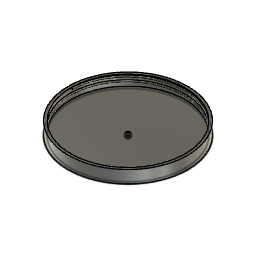
Container Lid (Autodesk Fusion 360 design; units mm, degrees)
Autodesk Fusion 360 part; units mm, degrees
sketch "Sketch1" plane through (0, 0, 0) normal (0, 0, 1) x (1, 0, 0)
  circle A0 centre (0, 0) radius 57.5
  circle A1 centre (0, 0) radius 55
  dimension "d1" = 115
  dimension "d2" = 110
  constraint coincident A0.centre A1.centre
  measures "d1" diameter of A0
  measures "d2" diameter of A1
extrude "Extrude2" add sketch "Sketch1" along normal blind 8 makes body 1
extrude "Extrude1" add sketch "Sketch1" along normal blind 3 separate body contours A1 makes body 2
extrude "Extrude3" add 1 faces at (56.2478, -5.5891, 8) along direction (0, 0, 1) blind 4 on bodies 1 bodies 1
extrude "Extrude4" cut 1 faces at (14.9005, 4.5962, 3) along direction (0, 0, -1) blind 1 on bodies 2 bodies 2
ref_plane "WorkPlane1" through (0, 0, 5) normal (0, 0, 1) x (1, 0, 0)
coil "CoilPrimitive1" add diameter 110 section circle size 1.5 on centre turns 1.5 pitch 4 right hand placed x (1, 0, 0) y (0, 1, 0) z (0, 0, 1) at (0, 0, 5) bodies 1
fillet "Fillet1" radius 0.7 2 edges at (-54.25, 0, 11) (54.25, 0, 5) on bodies 1
sketch "Sketch6" plane through (0, 0, 0) normal (0, 0, 1) x (1, 0, 0)
equation "d11 = 2 mm + 3 mm"
